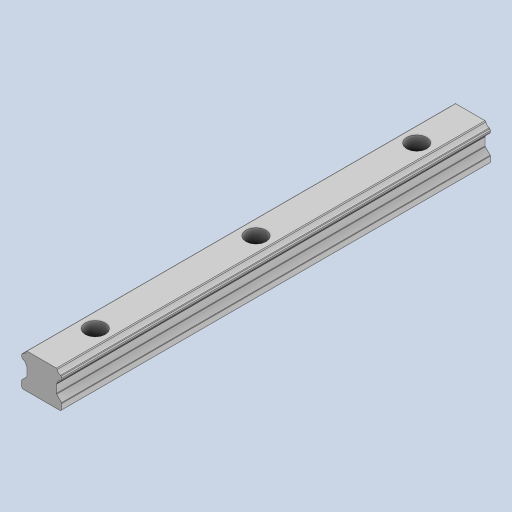
# Autodesk Inventor part: C-SV2R24-160_r
Saved by Autodesk Inventor 2023 (Build 270158000, 158)
## iProperties
Category: PARTsolutions
Company: MISUMI
Created: 2024-12-12
Part Number: C-SV2R24-160_r
Material: Generic
Catalog Web Link: www.cadenas.de
Description: C-SVR, C-SV2R, C-SVRL, C-SV2RL_rail-C-VALUE Linear Guides for Medium Load
Vendor: MISUMI
Document SubType Name: Modeling
Designer: psAdmin
Manufacturer: MISUMI
Mass: 25.7237 g
Surface Area: 100.566 cm^2
Volume: 25.7237 cm^3
Density: 1 g/cm^3
Appearance: PSOLRGB-175-175-175
PSOL_IDENT_0: {$CADENAS_DATA/23d-libs/misumi/metric/06_linear_guides/06_cn/c_svr/c_svr_rail.prj},210 {VTYP=3D},{NB=
PSOL_IDENT_1: C-SV2R24-160_r},{LINA=C-SV2R24-160},{NN=C-SVR, C-SV2R, C-SVRL, C-SV2RL_rail},{DATE=21.04.2022 05:41:
PSOL_IDENT_2: 22},{GEOMDATE=11.06.2020 07:59:11},{VERSION=},{LINEID=10},{WBVAR=NOB,LT,LS,ALT},{WBNUMERIC=LS}  {NB=
PSOL_IDENT_3: C-SV2R24-160_r},{LINA=C-SV2R24-160},{KT=DUMMY},{PN=C-SV2R24-160},{TYPE=C-SV},{H=24},{NOB=2},{LT=},{L
PSOL_IDENT_4: S=160},{LALG=[160,220,280,340,400,460,520,580,640,700,760,820,880,940,1000,1060,1120,1180,1240,1300,
PSOL_IDENT_5: 1360,1420,1480]},{LSALG=[160,220,280,340,400,460,520,580,640,700,760,820,880,940,1000,1060,1120,1180
PSOL_IDENT_6: ,1240,1300,1360,1420,1480]},{LALG0=[170:210/10],[230:270/10],[290:330/10],[350:390/10],[410:450/10],
PSOL_IDENT_7: [470:510/10],[530:570/10],[590:630/10],[650:690/10],[710:750/10],[770:810/10],[830:870/10],[890:930/
PSOL_IDENT_8: 10],[950:990/10],[1010:1050/10],[1070:1110/10],[1130:1170/10],[1190:1230/10],[1250:1290/10],[1310:13
PSOL_IDENT_9: 50/10],[1370:1410/10],[1430:1470/10]},{LMIN=170},{LMAX=1470},{W=34},{L1=39.3},{H1=13.0},{W1=15},{W2=
PSOL_IDENT_10: 9.5},{CAA=0.5},{DD1=4.5},{DD2=7.5},{HH=6.0},{DDH=4.5x7.5x6},{F=60},{G=20},{E=7},{LW1=7.217},{LW2=11.
PSOL_IDENT_11: 000},{LH1=8.221},{LH2=4.659},{LH3=3.221},{LH4=4.700},{LR1=1.431},{LR2=0.300},{LR3=0.300},{LR4=0.300}
PSOL_IDENT_12: ,{M=3},{ALT=},{ALTALG= '','N/A' },{NL=40},{CIFCP=40}
NB: C-SV2R24-160_r
NN: C-SVR, C-SV2R, C-SVRL, C-SV2RL_rail
NT: C-VALUE Linear Guides for Medium Load
NBSYN: $PN._r
LINA: C-SV2R24-160
CATALOG: Misumi
PN: C-SV2R24-160
H: 24
NOB: 2
LT: Selectable
LS: 160
W: 34
L1: 39.3
H1: 13
W1: 15
W2: 9.5
CAA: 0.5
DDH: 4.5x7.5x6
F: 60
G: 20
ALT: N/A
SUPPLIER: MISUMI
ARTICLENO: C-SV2R24-160_r
BOMINFO: C-SV2R24-160
CREATOR: CADENAS GmbH
Title: C-SV2R24-160
Author: Cadenas PARTsolutions
Comments: C-VALUE Linear Guides for Medium Load
Autodesk Inventor part; units mm, degrees
sketch "Sketch_2" plane through (0, 0, 0) normal (0, 0, 1) x (1, 0, 0)
  line L0 (-7.5, 10.787) -> (-7.5, 10.313)
  line L1 (-7.5, 10.313) -> (-7.2658, 9.8108)
  arc A0 (-7.2658, 9.8108) -> (-7.0326, 9.6401) centre (-6.9939, 9.9376) ccw
  arc A1 (-5.7891, 8.3153) -> (-7.0326, 9.6401) centre (-7.217, 8.221) ccw
  arc A2 (-5.7891, 8.3153) -> (-5.7019, 8.1229) centre (-5.4898, 8.335) ccw
  line L2 (-5.7019, 8.1229) -> (-5.5879, 8.0089)
  arc A3 (-5.5, 7.7967) -> (-5.5879, 8.0089) centre (-5.8, 7.7967) ccw
  line L3 (-5.5, 7.7967) -> (-5.5, 4.8243)
  arc A4 (-5.5879, 4.6121) -> (-5.5, 4.8243) centre (-5.8, 4.8243) ccw
  line L4 (-5.5879, 4.6121) -> (-7.4121, 2.7879)
  arc A5 (-7.4121, 2.7879) -> (-7.5, 2.5757) centre (-7.2, 2.5757) ccw
  line L5 (-7.5, 2.5757) -> (-7.5, 0.5)
  line L6 (-7.5, 0.5) -> (-7, 0)
  line L7 (-7, 0) -> (7, 0)
  line L8 (7, 0) -> (7.5, 0.5)
  line L9 (7.5, 0.5) -> (7.5, 2.5757)
  arc A6 (7.5, 2.5757) -> (7.4121, 2.7879) centre (7.2, 2.5757) ccw
  line L10 (7.4121, 2.7879) -> (5.5879, 4.6121)
  arc A7 (5.5, 4.8243) -> (5.5879, 4.6121) centre (5.8, 4.8243) ccw
  line L11 (5.5, 4.8243) -> (5.5, 7.7967)
  arc A8 (5.5879, 8.0089) -> (5.5, 7.7967) centre (5.8, 7.7967) ccw
  line L12 (5.5879, 8.0089) -> (5.7019, 8.1229)
  arc A9 (5.7019, 8.1229) -> (5.7891, 8.3153) centre (5.4898, 8.335) ccw
  arc A10 (7.0326, 9.6401) -> (5.7891, 8.3153) centre (7.217, 8.221) ccw
  arc A11 (7.0326, 9.6401) -> (7.2658, 9.8108) centre (6.9939, 9.9376) ccw
  line L13 (7.2658, 9.8108) -> (7.5, 10.313)
  line L14 (7.5, 10.313) -> (7.5, 10.787)
  line L15 (7.5, 10.787) -> (7.2653, 11.2903)
  arc A12 (7.2653, 11.2903) -> (7.0322, 11.461) centre (6.9934, 11.1635) ccw
  arc A13 (5.7938, 12.7312) -> (7.0322, 11.461) centre (7.217, 12.88) ccw
  arc A14 (5.7938, 12.7312) -> (5.4954, 13) centre (5.4954, 12.7) ccw
  line L16 (5.4954, 13) -> (-5.4954, 13)
  arc A15 (-5.4954, 13) -> (-5.7938, 12.7312) centre (-5.4954, 12.7) ccw
  arc A16 (-7.0322, 11.461) -> (-5.7938, 12.7312) centre (-7.217, 12.88) ccw
  arc A17 (-7.0322, 11.461) -> (-7.2653, 11.2903) centre (-6.9934, 11.1635) ccw
  line L17 (-7.2653, 11.2903) -> (-7.5, 10.787)
  constraints: 36 end point, 36 point on circle, 18 centre point
extrude "Extrusion1" add sketch "Sketch_2" along normal mid plane 160
sketch "Sketch2" plane through (-5.4954, 13, 80) normal (0, 1, 0) x (1, 0, 0)
  point P0 (5.4954, 20)
hole "Hole1" at (0, 13, 60) direction (0, -1, 0) diameter 4.5 depth 13 counterbore diameter 7.5 counterbore depth 6
pattern_linear "Rectangular Pattern1" count 3 spacing 60 along (0, 0, -1) of "Hole1"
ref_plane "to_block_1_XY" through (0, 13, 40) normal (0, 0, -1) x (1, 0, 0)
ref_plane "to_block_1_YZ" through (0, 13, 40) normal (1, 0, 0) x (0, -1, 0)
ref_plane "to_block_1_ZX" through (0, 13, 40) normal (0, -1, 0) x (0, 0, -1)
ref_plane "to_block_2_XY" through (0, 13, -40) normal (0, 0, 1) x (1, 0, 0)
ref_plane "to_block_2_YZ" through (0, 13, -40) normal (1, 0, 0) x (0, 1, 0)
ref_plane "to_block_2_ZX" through (0, 13, -40) normal (0, 1, 0) x (0, 0, 1)
body "Solid1"
